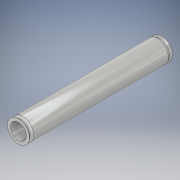
# Autodesk Inventor part: cilindar
Saved by Autodesk Inventor 2019 (Build 230136000, 136)
## iProperties
Created: 2018-11-25
Part Number: cilindar
Material: Aluminum 6061-AHC
Document SubType Name: Modeling
Designer: aleks
Density: 2.7 g/cm^3
Appearance: Aluminum - Dark
Author: aleks
Autodesk Inventor part; units mm, degrees
ref_plane "YZ Plane" through (0, 0, 0) normal (1, 0, 0) x (0, 1, 0)
ref_plane "XZ Plane" through (0, 0, 0) normal (0, 1, 0) x (-1, 0, 0)
ref_plane "XY Plane" through (0, 0, 0) normal (0, 0, 1) x (1, 0, 0)
sketch "Sketch1" plane through (0, 0, 0) normal (0, 1, 0) x (-1, 0, 0)
  line L0 (0, 68) -> (3, 68)
  line L1 (0, -68) -> (3, -68)
  line L2 (3, 64) -> (3, -64)
  line L3 (3, 68) -> (1.6451, 66.2542)
  arc A0 (1.6451, 66.2542) -> (3, 64) centre (3.1084, 65.5994) ccw
  line L4 (3, -68) -> (1.6451, -66.2542)
  arc A1 (3, -64) -> (1.6451, -66.2542) centre (3.1084, -65.5994) ccw
  line L5 (-7.5, 68) -> (-7.5, -52.2405)
  line L6 (0, 0) -> (0, -50)
  line L7 (0, -50) -> (0, 50)
  line L8 (0, -50) -> (-2.5, -50)
  line L9 (-2.5, -50) -> (-2.5, -52.5)
  line L10 (0, 50) -> (-2.5, 50)
  line L11 (-2.5, 50) -> (-2.5, 52.5)
  line L12 (-2.5, 52.5) -> (0, 52.5)
  line L13 (0, 68) -> (0, 52.5)
  line L14 (0, 50) -> (0, -50)
  line L15 (0, 0) -> (0, 50)
  line L16 (0, 52.5) -> (0, 64)
  line L17 (-2.5, -52.5) -> (0, -52.5)
  line L18 (0, -52.5) -> (0, -68)
  point P0 (-3, -64)
  dimension "d15" = 3
  dimension "d16" = 7.5
  constraints: 38 end point, 5 horizontal, 4 point on circle, 2 centre point, 2 perpendicular, 2 vertical, 1 point on line
  measures "d15" distance between parallel lines of L2 L7
  measures "d16" distance between parallel lines of L5 L7
revolve "Revolution1" add sketch "Sketch1" angle 360 about axis through (7.5, 0, 68) along (0, 0, -1)
body "Solid1"
